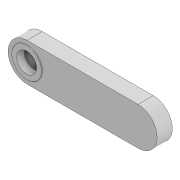
# Autodesk Inventor part: HMI arm bewegende deel
Saved by Autodesk Inventor 2020.3 (Build 243373000, 373)
## iProperties
Created: 2020-12-03
Part Number: HMI arm bewegende deel
Material: Generic
Document SubType Name: Modeling
Designer: Svend
Density: 1 g/cm^3
Appearance: Default
Author: Svend
Autodesk Inventor part; units mm, degrees
ref_plane "YZ Plane" through (0, 0, 0) normal (1, 0, 0) x (0, 1, 0)
ref_plane "XZ Plane" through (0, 0, 0) normal (0, 1, 0) x (-1, 0, 0)
ref_plane "XY Plane" through (0, 0, 0) normal (0, 0, 1) x (1, 0, 0)
sketch "Sketch1" plane through (0, 0, 0) normal (0, 0, 1) x (1, 0, 0)
  circle A0 centre (0, 0) radius 25
  circle A1 centre (-146, 0) radius 25
  line L0 (-146, 25) -> (0, 25)
  line L1 (-146, -25) -> (0, -25)
  point P0 (-171, 0)
  point P1 (25, 0)
  dimension "d0" = 50
  dimension "d1" = 196
  constraints: 6 point on circle, 4 end point, 4 tangent, 3 horizontal alignment, 2 centre point, 1 coincident, 1 equal radius
  measures "d0" diameter of A0
  measures "d1" distance of point (-171, 0) point (25, 0)
extrude "Extrusion1" add sketch "Sketch1" along normal blind 20
sketch "Sketch2" plane through (0, 0, 20) normal (0, 0, 1) x (1, 0, 0)
  arc A0 (0, -25) -> (0, 25) centre (0, 0) ccw projected
  line L0 (0, 25) -> (-146, 25) projected
  arc A1 (-146, 25) -> (-146, -25) centre (-146, 0) ccw projected
  line L1 (-146, -25) -> (0, -25) projected
  circle A2 centre (-146, 0) radius 20
  dimension "d4" = 40
  constraints: 1 centre point, 1 coincident
  measures "d4" diameter of A2
extrude "Extrusion2" add sketch "Sketch2" along normal blind 0.5 contours A2
chamfer "Chamfer1" distance 0.5 angle 45 1 edges at (-166, 0, 20.5)
sketch "Sketch3" plane through (-146, 0, 20.5) normal (0, 0, 1) x (1, 0, 0)
  circle A0 centre (0, 0) radius 20 projected
  arc A1 (146, -25) -> (146, 25) centre (146, 0) ccw projected
  line L0 (146, 25) -> (0, 25) projected
  arc A2 (0, 25) -> (0, -25) centre (0, 0) ccw projected
  line L1 (0, -25) -> (146, -25) projected
  circle A3 centre (0, 0) radius 13
  dimension "d10" = 26
  constraints: 1 centre point, 1 coincident
  measures "d10" diameter of A3
extrude "Extrusion3" cut sketch "Sketch3" against normal blind 10 contours A3
body "Solid1"
